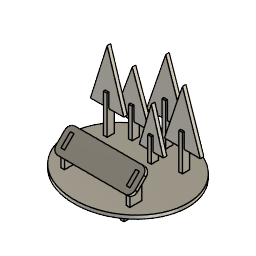
lasercutting v14 (Autodesk Fusion 360 design; units mm, degrees)
Autodesk Fusion 360 part; units mm, degrees
(part 1 of 2)
sketch "Sketch1" plane through (0, 0, 0) normal (0, 0, 1) x (1, 0, 0)
  circle A0 centre (0, 25) radius 50 construction
  ellipse E0 centre (0, 25) end of major axis (-50, 25) minor radius 45
  line L0 (50, 25) -> (-50, 25) construction
  line L1 (0, 70) -> (0, -20) construction
  dimension "d3" = 100
  constraint coincident E0 L0.start
  constraint coincident E0 L0.end
  constraint coincident E0 L1.start
  constraint coincident E0 L1.end
  constraint concentric A0 E0
  constraint horizontal L0
  measures "d3" diameter of A0
extrude "Extrude1" add sketch "Sketch1" along normal blind 3 makes body 1
sketch "Sketch2" plane through (0, 0, 3) normal (0, 0, 1) x (-1, 0, 0)
  line L0 (28.8477, -7.7401) -> (25.8477, -7.7401)
  line L1 (25.8477, -7.7401) -> (25.8477, 2.2599)
  line L2 (25.8477, 2.2599) -> (28.8477, 2.2599)
  line L3 (28.8477, 2.2599) -> (28.8477, -7.7401)
  line L4 (0, -100) -> (0, 100) construction
  line L5 (-28.8477, -7.7401) -> (-25.8477, -7.7401)
  line L6 (-25.8477, -7.7401) -> (-25.8477, 2.2599)
  line L7 (-28.8477, 2.2599) -> (-28.8477, -7.7401)
  line L8 (-25.8477, 2.2599) -> (-28.8477, 2.2599)
  ellipse E0 centre (0, -25) end of major axis (50, -25) minor radius 45
  dimension "d6" = 3
  constraint horizontal L0
  constraint vertical L1
  constraint horizontal L2
  constraint vertical L3
  constraint vertical L4
  constraint symmetric L0.start L4 L5.start
  constraint symmetric L0.end L4 L5.end
  constraint symmetric L1.end L4 L6.end
  constraint symmetric L2.end L4 L7.start
  measures "d6" distance of L0.start L0.end
extrude "Extrude2" add sketch "Sketch2" along normal blind 20 separate body contours L0 L1 L2 L3 | L5 L6 L7 L8 makes body 2 at (-25.8477, 4.4068, 9.6667) makes body 3 at (28.8477, 1.0734, 9.6667)
extrude "Extrude3" add sketch "Sketch2" against normal blind 8 contours L0 L1 L2 L3 | L5 L6 L7 L8 bodies 2 3
sketch "Sketch3" plane through (0, -2.2599, 0) normal (0, -1, 0) x (1, 0, 0)
  line L0 (-25.8477, -5) -> (-25.8477, 23)
  line L1 (-25.8477, 23) -> (-28.8477, 23)
  line L2 (-28.8477, 23) -> (-28.8477, -5)
  line L3 (-28.8477, -5) -> (-25.8477, -5)
  line L4 (0, 15) -> (0, -10) construction
  line L5 (-28.8477, 0.0164) -> (-25.8477, 0.0164)
  line L6 (-25.8477, 0.0164) -> (-25.8477, -5)
  line L7 (-25.8477, -5) -> (-28.8477, -5)
  line L8 (-28.8477, -5) -> (-28.8477, 0.0164)
  line L9 (28.8477, 0.0164) -> (25.8477, 0.0164)
  line L10 (28.8477, -5) -> (28.8477, 0.0164)
  line L11 (25.8477, -5) -> (28.8477, -5)
  line L12 (25.8477, 0.0164) -> (25.8477, -5)
  constraint vertical L4
  constraint horizontal L5
  constraint vertical L6
  constraint horizontal L7
  constraint vertical L8
  constraint coincident L0.start L3.end
  constraint coincident L2 L5.start
  constraint symmetric L4 L5.start L9.start
  constraint symmetric L4 L5.end L9.end
  constraint symmetric L4 L0.start L11.start
  constraint symmetric L4 L2.end L10.start
extrude "Extrude4" add sketch "Sketch3" along normal blind 5 contours L0 L2 L3 L5 L6 L7 L8 | L9 L10 L11 L12 bodies 2 3
extrude "Extrude5" add sketch "Sketch3" against normal blind 5 from surface at -10 contours L0 L2 L3 L5 L6 L7 L8 | L9 L10 L11 L12 bodies 2 3
chamfer "Chamfer1" distance 10 angle 45 2 edges at (27.3477, -2.2599, 23) (-27.3477, -2.2599, 23) on bodies 2 3
extrude "Extrude6" add 2 faces at (-26.8477, 7.7388, 23) (-26.8477, 1.0728, 16.3347) along direction (0, -0.707107, 0.707107) blind 3 separate body on bodies 2 makes body 4
move_face "OffsetFaces1" offset -3 1 faces at (-26.8477, -2.967, 13.7091) on bodies 4
mirror "Mirror1" about plane through (0, 0, 0) normal (1, 0, 0) of bodies 4 makes body 5
combine "Combine1" operation add target body 4 tool bodies 2 5 3 makes body 6 at (28.8477, 5.1139, 12.7132)
sketch "Sketch5" plane through (0, -9.7513, 9.7513) normal (0, -0.707107, 0.707107) x (1, 0, 0)
  line L0 (-25.8477, 10.5944) -> (-25.8477, 21.7365)
  line L1 (-25.8477, 21.7365) -> (-28.8477, 21.7365)
  line L2 (-28.8477, 21.7365) -> (-28.8477, 10.5944)
  line L3 (-28.8477, 10.5944) -> (-25.8477, 10.5944)
  line L4 (0, 4) -> (0, -46) construction
  line L5 (0, 25.9792) -> (0, 5.8372)
  line L6 (0, 5.8372) -> (-28, 5.8372)
  line L7 (-33, 10.8372) -> (-33, 20.9792)
  line L8 (-28, 25.9792) -> (0, 25.9792)
  arc A0 (-28, 25.9792) -> (-33, 20.9792) centre (-28, 20.9792) ccw
  arc A1 (-33, 10.8372) -> (-28, 5.8372) centre (-28, 10.8372) ccw
  dimension "d24" = 5
  constraint vertical L4
  constraint vertical L5
  constraint tangent L7 A0
  constraint tangent L8 A0
  constraint tangent L6 A1
  constraint tangent L7 A1
  constraint equal A0 A1
  measures "d24" radius of A0
extrude "Extrude7" add sketch "Sketch5" against normal blind 3 separate body makes body 7
mirror "Mirror2" about plane through (0, 0, 0) normal (1, 0, 0) of bodies 7 merged
sketch "Sketch6" plane through (0, 0, 3) normal (0, 0, 1) x (-1, 0, 0)
  line L0 (-1.5, -55) -> (1.5, -55)
  line L1 (1.5, -55) -> (1.5, -61)
  line L2 (1.5, -61) -> (-1.5, -61)
  line L3 (-1.5, -61) -> (-1.5, -55)
  line L4 (-1.5, -55) -> (1.5, -61) construction
  line L5 (1.5, -55) -> (-1.5, -61) construction
  line L6 (18.5, -47) -> (21.5, -47)
  line L7 (21.5, -47) -> (21.5, -53)
  line L8 (21.5, -53) -> (18.5, -53)
  line L9 (18.5, -53) -> (18.5, -47)
  line L10 (18.5, -47) -> (21.5, -53) construction
  line L11 (21.5, -47) -> (18.5, -53) construction
  line L12 (-23.5, -44) -> (-26.5, -44)
  line L13 (-26.5, -44) -> (-26.5, -50)
  line L14 (-26.5, -50) -> (-23.5, -50)
  line L15 (-23.5, -50) -> (-23.5, -44)
  line L16 (-23.5, -44) -> (-26.5, -50) construction
  line L17 (-26.5, -44) -> (-23.5, -50) construction
  line L18 (-6.5, -38) -> (-3.5, -38)
  line L19 (-3.5, -38) -> (-3.5, -44)
  line L20 (-3.5, -44) -> (-6.5, -44)
  line L21 (-6.5, -44) -> (-6.5, -38)
  line L22 (-6.5, -38) -> (-3.5, -44) construction
  line L23 (-3.5, -38) -> (-6.5, -44) construction
  line L24 (31.5, -39) -> (34.5, -39)
  line L25 (34.5, -39) -> (34.5, -45)
  line L26 (34.5, -45) -> (31.5, -45)
  line L27 (31.5, -45) -> (31.5, -39)
  line L28 (31.5, -39) -> (34.5, -45) construction
  line L29 (34.5, -39) -> (31.5, -45) construction
  ellipse E0 centre (0, -25) end of major axis (50, -25) minor radius 45
  point P0 (0, -58)
  point P1 (20, -50)
  point P2 (-25, -47)
  point P3 (-5, -41)
  point P4 (33, -42)
  dimension "d29" = 3
  dimension "d30" = 6
  dimension "d49" = 3
  dimension "d50" = 3
  dimension "d51" = 6
  dimension "d52" = 3
  dimension "d53" = 3
  dimension "d54" = 6
  constraint horizontal L0
  constraint perpendicular L0 L1
  constraint parallel L0 L2
  constraint parallel L1 L3
  constraint coincident L4 P0
  constraint coincident L5 P0
  constraint horizontal L6
  constraint perpendicular L6 L7
  constraint parallel L6 L8
  constraint parallel L7 L9
  constraint coincident L10 P1
  constraint coincident L11 P1
  constraint horizontal L12
  constraint perpendicular L12 L13
  constraint parallel L12 L14
  constraint parallel L13 L15
  constraint coincident L16 P2
  constraint coincident L17 P2
  constraint horizontal L18
  constraint perpendicular L18 L19
  constraint parallel L18 L20
  constraint parallel L19 L21
  constraint coincident L22 P3
  constraint coincident L23 P3
  constraint horizontal L24
  constraint perpendicular L24 L25
  constraint parallel L24 L26
  constraint parallel L25 L27
  constraint coincident L28 P4
  constraint coincident L29 P4
  measures "d29" distance of L1.end L2.end
  measures "d30" distance of L0.end L1.end
  measures "d49" distance of L7.end L8.end
  measures "d50" distance of L13.end L14.end
  measures "d51" distance of L12.end L13.end
  measures "d52" distance of L19.end L20.end
  measures "d53" distance of L25.end L26.end
  measures "d54" distance of L24.end L25.end
extrude "Extrude8" add sketch "Sketch6" along normal blind 35 separate body contours L0 L1 L2 L3 makes body 8
sketch "Sketch7" plane through (-1.5, 0, 0) normal (-1, 0, 0) x (0, -1, 0)
  line L0 (-55, 3) -> (-55, 38)
  line L1 (-55, 38) -> (-61, 38)
  line L2 (-61, 38) -> (-61, 3)
  line L3 (-59.5, 33) -> (-56.5, 33)
  line L4 (-56.5, 33) -> (-56.5, 43)
  line L5 (-56.5, 43) -> (-59.5, 43)
  line L6 (-59.5, 43) -> (-59.5, 33)
  line L7 (-59.5, 33) -> (-56.5, 43) construction
  line L8 (-56.5, 33) -> (-59.5, 43) construction
  line L9 (-61, 3) -> (-55, 3)
  point P0 (-58, 38)
  dimension "d33" = 3
  dimension "d34" = 10
  constraint horizontal L3
  constraint perpendicular L3 L4
  constraint parallel L3 L5
  constraint parallel L4 L6
  constraint coincident L7 P0
  constraint coincident L8 P0
  constraint midpoint L1 P0
  measures "d33" distance of L4.end L5.end
  measures "d34" distance of L3.end L4.end
extrude "Extrude9" cut sketch "Sketch7" against normal blind 3 contours L1 L3 L4 L6 bodies 1 8
extrude "Extrude10" add sketch "Sketch6" against normal blind 8 contours L0 L1 L2 L3 bodies 8
sketch "Sketch8" plane through (0, 61, 0) normal (0, 1, 0) x (-1, 0, 0)
  line L0 (1.5, -5) -> (1.5, 38)
  line L1 (1.5, 38) -> (-1.5, 38)
  line L2 (-1.5, 38) -> (-1.5, -5)
  line L3 (-1.5, -5) -> (1.5, -5)
  line L4 (-1.5, 0) -> (1.5, 0)
  line L5 (1.5, 0) -> (1.5, -5)
  line L6 (1.5, -5) -> (-1.5, -5)
  line L7 (-1.5, -5) -> (-1.5, 0)
  constraint horizontal L4
  constraint vertical L5
  constraint horizontal L6
  constraint vertical L7
  constraint coincident L0.start L3.end
  constraint coincident L2 L4.start
extrude "Extrude11" add sketch "Sketch8" along normal blind 5 contours L0 L2 L3 L4 L5 L6 L7 bodies 8
extrude "Extrude12" add sketch "Sketch8" against normal blind 11 contours L0 L2 L3 L4 L5 L6 L7 bodies 8
sketch "Sketch9" plane through (0, 59.5, 0) normal (0, -1, 0) x (1, 0, 0)
  line L0 (-1.5, 38) -> (-1.5, 33)
  line L1 (-1.5, 33) -> (1.5, 33)
  line L2 (1.5, 33) -> (1.5, 38)
  line L3 (1.5, 38) -> (-1.5, 38)
  line L4 (-6, 38) -> (5.5, 38) construction
  line L5 (-6.5, 33) -> (5.7756, 33) construction
  line L6 (0, 70) -> (-16.0582, 22.6488)
  line L7 (-1.5, 38) -> (-1.5, 16) construction
  line L8 (-16.0582, 22.6488) -> (-1.5, 22.6488)
  line L9 (-1.5, 33) -> (-1.5, 22.6488)
  line L10 (0, 85) -> (0, 0) construction
  line L11 (0, 70) -> (16.0582, 22.6488)
  line L12 (16.0582, 22.6488) -> (1.5, 22.6488)
  line L13 (1.5, 33) -> (1.5, 22.6488)
  line L14 (-1.5, 33) -> (1.5, 33)
  dimension "d45" = 5
  dimension "d46" = 50
  constraint perpendicular L2 L4
  constraint perpendicular L0 L5
  constraint coincident L0.start L3.end
  constraint perpendicular L5 L7
  constraint coincident L7 L8.end
  constraint perpendicular L7 L8
  constraint coincident L0.end L1.start
  constraint coincident L10.end origin
  constraint perpendicular L8 L10
  constraint symmetric L6.start L10 L11.start
  constraint symmetric L6.end L10 L11.end
  constraint symmetric L8.end L10 L12.end
  constraint symmetric L0.end L10 L1.end
  measures "d45" distance of L4 L5
  measures "d46" distance of L6.start L6.end
extrude "Extrude13" add sketch "Sketch9" along normal blind 3 separate body contours L0 L2 L3 L6 L8 L9 L11 L12 L13 makes body 9
extrude "Extrude14" add sketch "Sketch6" along normal blind 25 separate body contours L6 L7 L8 L9 makes body 10
extrude "Extrude15" add sketch "Sketch6" against normal blind 8 contours L6 L7 L8 L9 bodies 10
sketch "Sketch10" plane through (0, 47, 0) normal (0, -1, 0) x (1, 0, 0)
  line L0 (-18.5, -5) -> (-18.5, 28)
  line L1 (-18.5, 28) -> (-21.5, 28)
  line L2 (-21.5, 28) -> (-21.5, -5)
  line L3 (-21.5, -5) -> (-18.5, -5)
  line L4 (-21.5, 0) -> (-18.5, 0)
  line L5 (-18.5, 0) -> (-18.5, -5)
  line L6 (-18.5, -5) -> (-21.5, -5)
  line L7 (-21.5, -5) -> (-21.5, 0)
  constraint horizontal L4
  constraint vertical L5
  constraint horizontal L6
  constraint vertical L7
  constraint coincident L0.start L3.end
  constraint coincident L2 L4.start
extrude "Extrude16" add sketch "Sketch10" along normal blind 5 contours L0 L2 L3 L4 L5 L6 L7 bodies 10
extrude "Extrude17" add sketch "Sketch10" against normal blind 11 contours L0 L2 L3 L4 L5 L6 L7 bodies 10
sketch "Sketch11" plane through (-21.5, 0, 0) normal (-1, 0, 0) x (0, -1, 0)
  line L0 (-47, 0) -> (-47, 28)
  line L1 (-47, 28) -> (-53, 28)
  line L2 (-53, 28) -> (-53, 0)
  line L3 (-53, 0) -> (-58, 0)
  line L4 (-58, 0) -> (-58, -5)
  line L5 (-58, -5) -> (-42, -5)
  line L6 (-42, -5) -> (-42, 0)
  line L7 (-42, 0) -> (-47, 0)
  line L8 (-48.5, 33) -> (-51.5, 33)
  line L9 (-51.5, 33) -> (-51.5, 23)
  line L10 (-51.5, 23) -> (-48.5, 23)
  line L11 (-48.5, 23) -> (-48.5, 33)
  line L12 (-48.5, 33) -> (-51.5, 23) construction
  line L13 (-51.5, 33) -> (-48.5, 23) construction
  point P0 (-50, 28)
  dimension "d63" = 3
  dimension "d64" = 10
  constraint horizontal L8
  constraint perpendicular L8 L9
  constraint parallel L8 L10
  constraint parallel L9 L11
  constraint coincident L12 P0
  constraint coincident L13 P0
  constraint midpoint L1 P0
  measures "d63" distance of L9.end L10.end
  measures "d64" distance of L8.end L9.end
extrude "Extrude18" cut sketch "Sketch11" against normal blind 3 contours L1 L9 L10 L11 bodies 10
sketch "Sketch12" plane through (0, 51.5, 0) normal (0, -1, 0) x (1, 0, 0)
  line L0 (-21.5, 28) -> (-21.5, 23)
  line L1 (-21.5, 23) -> (-18.5, 23)
  line L2 (-18.5, 23) -> (-18.5, 28)
  line L3 (-18.5, 28) -> (-21.5, 28)
  line L4 (-24.1, 28) -> (-15.2, 28) construction
  line L5 (-23.9, 23) -> (-15.1, 23) construction
  line L6 (-20, 55) -> (-34, 16)
  line L7 (-21.5, 28) -> (-21.5, 10) construction
  line L8 (-34, 16) -> (-21.5, 16)
  line L9 (-21.5, 16) -> (-21.5, 23)
  line L10 (-21.5, 23) -> (-20, 23)
  line L11 (-20, 59) -> (-20, 5) construction
  line L12 (-20, 55) -> (-6, 16)
  line L13 (-6, 16) -> (-18.5, 16)
  line L14 (-18.5, 16) -> (-18.5, 23)
  line L15 (-18.5, 23) -> (-20, 23)
  dimension "d67" = 5
  constraint perpendicular L2 L4
  constraint perpendicular L2 L5
  constraint coincident L0.start L3.end
  constraint perpendicular L4 L7
  constraint coincident L7 L8.end
  constraint perpendicular L7 L8
  constraint coincident L0.end L1.start
  constraint midpoint L1 L10.end
  constraint perpendicular L10 L11
  constraint symmetric L6.start L11 L12.start
  constraint symmetric L6.end L11 L12.end
  constraint symmetric L8.end L11 L13.end
  constraint symmetric L0.end L11 L1.end
  constraint symmetric L10.end L11 L15.end
  measures "d67" distance of L4 L5
extrude "Extrude19" add sketch "Sketch12" along normal blind 3 separate body contours L0 L2 L3 L6 L8 L9 L12 L13 L14 makes body 11
extrude "Extrude20" add sketch "Sketch6" along normal blind 30 separate body contours L12 L13 L14 L15 makes body 12
extrude "Extrude21" add sketch "Sketch6" against normal blind 8 contours L12 L13 L14 L15 bodies 12
sketch "Sketch13" plane through (0, 44, 0) normal (0, -1, 0) x (1, 0, 0)
  line L0 (26.5, -5) -> (26.5, 33)
  line L1 (26.5, 33) -> (23.5, 33)
  line L2 (23.5, 33) -> (23.5, -5)
  line L3 (23.5, -5) -> (26.5, -5)
  line L4 (23.5, 0) -> (26.5, 0)
  line L5 (26.5, 0) -> (26.5, -5)
  line L6 (26.5, -5) -> (23.5, -5)
  line L7 (23.5, -5) -> (23.5, 0)
  constraint horizontal L4
  constraint vertical L5
  constraint horizontal L6
  constraint vertical L7
  constraint coincident L0.start L3.end
  constraint coincident L2 L4.start
extrude "Extrude22" add sketch "Sketch13" along normal blind 5 contours L0 L2 L3 L4 L5 L6 L7 bodies 12
extrude "Extrude23" add sketch "Sketch13" against normal blind 11 contours L0 L2 L3 L4 L5 L6 L7 bodies 12
sketch "Sketch14" plane through (26.5, 0, 0) normal (1, 0, 0) x (0, 1, 0)
  line L0 (50, 0) -> (50, 33)
  line L1 (50, 33) -> (44, 33)
  line L2 (44, 33) -> (44, 0)
  line L3 (44, 0) -> (39, 0)
  line L4 (39, 0) -> (39, -5)
  line L5 (39, -5) -> (55, -5)
  line L6 (55, -5) -> (55, 0)
  line L7 (55, 0) -> (50, 0)
  line L8 (45.5, 28) -> (48.5, 28)
  line L9 (48.5, 28) -> (48.5, 38)
  line L10 (48.5, 38) -> (45.5, 38)
  line L11 (45.5, 38) -> (45.5, 28)
  line L12 (45.5, 28) -> (48.5, 38) construction
  line L13 (48.5, 28) -> (45.5, 38) construction
  point P0 (47, 33)
  dimension "d78" = 3
  dimension "d79" = 10
  constraint horizontal L8
  constraint perpendicular L8 L9
  constraint parallel L8 L10
  constraint parallel L9 L11
  constraint coincident L12 P0
  constraint coincident L13 P0
  constraint midpoint L1 P0
  measures "d78" distance of L9.end L10.end
  measures "d79" distance of L8.end L9.end
extrude "Extrude24" cut sketch "Sketch14" against normal blind 3 contours L1 L8 L9 L11 bodies 12
sketch "Sketch15" plane through (0, 48.5, 0) normal (0, -1, 0) x (1, 0, 0)
  line L0 (26.5, 28) -> (26.5, 33)
  line L1 (26.5, 33) -> (23.5, 33)
  line L2 (23.5, 33) -> (23.5, 28)
  line L3 (23.5, 28) -> (26.5, 28)
  line L4 (20.7463, 33) -> (31.5, 33) construction
  line L5 (20.7463, 28) -> (31.5, 28) construction
  line L6 (23.5, 35) -> (23.5, 13) construction
  line L7 (25, 57) -> (25, 12) construction
  line L8 (25, 65) -> (10, 20)
  line L9 (10, 20) -> (23.5, 20)
  line L10 (23.5, 20) -> (23.5, 28)
  line L11 (23.5, 28) -> (25, 28)
  line L12 (25, 65) -> (40, 20)
  line L13 (40, 20) -> (26.5, 20)
  line L14 (26.5, 20) -> (26.5, 28)
  line L15 (26.5, 28) -> (25, 28)
  dimension "d82" = 5
  constraint perpendicular L0 L4
  constraint parallel L4 L5
  constraint perpendicular L5 L6
  constraint perpendicular L5 L7
  constraint coincident L6 L9.end
  constraint perpendicular L6 L9
  constraint coincident L2.end L3.start
  constraint midpoint L3 L11.end
  constraint symmetric L7 L8.start L12.start
  constraint symmetric L7 L8.end L12.end
  constraint symmetric L7 L9.end L13.end
  constraint symmetric L7 L2.end L0.start
  constraint symmetric L7 L11.end L15.end
  measures "d82" distance of L4 L5
extrude "Extrude25" add sketch "Sketch15" along normal blind 3 separate body contours L0 L1 L2 L8 L9 L10 L12 L13 L14 makes body 13
extrude "Extrude26" add sketch "Sketch6" along normal blind 32 separate body contours L24 L25 L26 L27 makes body 14
extrude "Extrude27" add sketch "Sketch6" against normal blind 8 contours L24 L25 L26 L27 bodies 14
sketch "Sketch16" plane through (0, 39, 0) normal (0, -1, 0) x (1, 0, 0)
  line L0 (-31.5, -5) -> (-31.5, 35)
  line L1 (-31.5, 35) -> (-34.5, 35)
  line L2 (-34.5, 35) -> (-34.5, -5)
  line L3 (-34.5, -5) -> (-31.5, -5)
  line L4 (-34.5, 0) -> (-31.5, 0)
  line L5 (-31.5, 0) -> (-31.5, -5)
  line L6 (-31.5, -5) -> (-34.5, -5)
  line L7 (-34.5, -5) -> (-34.5, 0)
  constraint horizontal L4
  constraint vertical L5
  constraint horizontal L6
  constraint vertical L7
  constraint coincident L0.start L3.end
  constraint coincident L2 L4.start
extrude "Extrude28" add sketch "Sketch16" along normal blind 5 contours L0 L2 L3 L4 L5 L6 L7 bodies 14
extrude "Extrude29" add sketch "Sketch16" against normal blind 11 contours L0 L2 L3 L4 L5 L6 L7 bodies 14
sketch "Sketch17" plane through (-34.5, 0, 0) normal (-1, 0, 0) x (0, -1, 0)
  line L0 (-39, 0) -> (-39, 35)
  line L1 (-39, 35) -> (-45, 35)
  line L2 (-45, 35) -> (-45, 0)
  line L3 (-45, 0) -> (-50, 0)
  line L4 (-50, 0) -> (-50, -5)
  line L5 (-50, -5) -> (-34, -5)
  line L6 (-34, -5) -> (-34, 0)
  line L7 (-34, 0) -> (-39, 0)
  line L8 (-40.5, 40) -> (-43.5, 40)
  line L9 (-43.5, 40) -> (-43.5, 30)
  line L10 (-43.5, 30) -> (-40.5, 30)
  line L11 (-40.5, 30) -> (-40.5, 40)
  line L12 (-40.5, 40) -> (-43.5, 30) construction
  line L13 (-43.5, 40) -> (-40.5, 30) construction
  point P0 (-42, 35)
  dimension "d93" = 3
  dimension "d94" = 10
  constraint horizontal L8
  constraint perpendicular L8 L9
  constraint parallel L8 L10
  constraint parallel L9 L11
  constraint coincident L12 P0
  constraint coincident L13 P0
  constraint midpoint L1 P0
  measures "d93" distance of L9.end L10.end
  measures "d94" distance of L8.end L9.end
extrude "Extrude30" cut sketch "Sketch17" against normal blind 3 contours L1 L9 L10 L11 bodies 14
sketch "Sketch18" plane through (0, 43.5, 0) normal (0, -1, 0) x (1, 0, 0)
  line L0 (-34.5, 35) -> (-34.5, 30)
  line L1 (-34.5, 30) -> (-31.5, 30)
  line L2 (-31.5, 30) -> (-31.5, 35)
  line L3 (-31.5, 35) -> (-34.5, 35)
  line L4 (-38, 35) -> (-29, 35) construction
  line L5 (-38.4345, 30) -> (-28.5, 30) construction
  line L6 (-34.5, 36.4776) -> (-34.5, 15.5578) construction
  line L7 (-33, 73) -> (-33, 8) construction
  line L8 (-33, 68) -> (-47, 23)
  line L9 (-47, 23) -> (-34.5, 23)
  line L10 (-34.5, 23) -> (-34.5, 30)
  line L11 (-34.5, 30) -> (-33, 30)
  line L12 (-33, 68) -> (-19, 23)
  line L13 (-19, 23) -> (-31.5, 23)
  line L14 (-31.5, 23) -> (-31.5, 30)
  line L15 (-31.5, 30) -> (-33, 30)
  dimension "d97" = 5
  constraint perpendicular L0 L4
  constraint horizontal L5
  constraint perpendicular L5 L6
  constraint perpendicular L5 L7
  constraint coincident L7 L8.start
  constraint coincident L6 L9.end
  constraint perpendicular L6 L9
  constraint coincident L0.end L1.start
  constraint perpendicular L5 L10
  constraint midpoint L1 L11.end
  constraint symmetric L7 L8.start L12.start
  constraint symmetric L7 L8.end L12.end
  constraint symmetric L7 L9.end L13.end
  constraint symmetric L7 L0.end L1.end
  constraint symmetric L7 L11.end L15.end
  measures "d97" distance of L4 L5
extrude "Extrude31" add sketch "Sketch18" along normal blind 3 separate body contours L0 L2 L3 L8 L9 L10 L12 L13 L14 makes body 15
extrude "Extrude32" add sketch "Sketch6" along normal blind 20 separate body contours L18 L19 L20 L21 makes body 16
extrude "Extrude33" add sketch "Sketch6" against normal blind 8 contours L18 L19 L20 L21 bodies 16
sketch "Sketch19" plane through (0, 38, 0) normal (0, -1, 0) x (1, 0, 0)
  line L0 (6.5, -5) -> (6.5, 23)
  line L1 (6.5, 23) -> (3.5, 23)
  line L2 (3.5, 23) -> (3.5, -5)
  line L3 (3.5, -5) -> (6.5, -5)
  line L4 (3.5, 0) -> (6.5, 0)
  line L5 (6.5, 0) -> (6.5, -5)
  line L6 (6.5, -5) -> (3.5, -5)
  line L7 (3.5, -5) -> (3.5, 0)
  constraint horizontal L4
  constraint vertical L5
  constraint horizontal L6
  constraint vertical L7
  constraint coincident L0.start L3.end
  constraint coincident L2 L4.start
extrude "Extrude34" add sketch "Sketch19" along normal blind 5 contours L0 L2 L3 L4 L5 L6 L7 bodies 16
extrude "Extrude35" add sketch "Sketch19" against normal blind 11 contours L0 L2 L3 L4 L5 L6 L7 bodies 16
sketch "Sketch20" plane through (6.5, 0, 0) normal (1, 0, 0) x (0, 1, 0)
  line L0 (44, 0) -> (44, 23)
  line L1 (44, 23) -> (38, 23)
  line L2 (38, 23) -> (38, 0)
  line L3 (38, 0) -> (33, 0)
  line L4 (33, 0) -> (33, -5)
  line L5 (33, -5) -> (49, -5)
  line L6 (49, -5) -> (49, 0)
  line L7 (49, 0) -> (44, 0)
  line L8 (39.5, 18) -> (42.5, 18)
  line L9 (42.5, 18) -> (42.5, 28)
  line L10 (42.5, 28) -> (39.5, 28)
  line L11 (39.5, 28) -> (39.5, 18)
  line L12 (39.5, 18) -> (42.5, 28) construction
  line L13 (42.5, 18) -> (39.5, 28) construction
  point P0 (41, 23)
  dimension "d108" = 3
  dimension "d109" = 10
  constraint horizontal L8
  constraint perpendicular L8 L9
  constraint parallel L8 L10
  constraint parallel L9 L11
  constraint coincident L12 P0
  constraint coincident L13 P0
  constraint midpoint L1 P0
  measures "d108" distance of L9.end L10.end
  measures "d109" distance of L8.end L9.end
extrude "Extrude36" cut sketch "Sketch20" against normal blind 3 contours L1 L8 L9 L11 bodies 16
sketch "Sketch21" plane through (0, 42.5, 0) normal (0, -1, 0) x (1, 0, 0)
  line L0 (6.5, 18) -> (6.5, 23)
  line L1 (6.5, 23) -> (3.5, 23)
  line L2 (3.5, 23) -> (3.5, 18)
  line L3 (3.5, 18) -> (6.5, 18)
  line L4 (1.5, 23) -> (12.5, 23) construction
  line L5 (3.5, 28.0693) -> (3.5, 5) construction
  line L6 (5, 68.4762) -> (5, -10) construction
  line L7 (5, 45) -> (-5, 11)
  line L8 (-5, 11) -> (3.5, 11)
  line L9 (3.5, 11) -> (3.5, 18)
  line L10 (3.5, 18) -> (5, 18)
  line L11 (5, 45) -> (15, 11)
  line L12 (6.5, 11) -> (6.5, 18)
  line L13 (6.5, 18) -> (5, 18)
  line L14 (15, 11) -> (6.5, 11)
  constraint perpendicular L2 L4
  constraint perpendicular L1 L5
  constraint coincident L6 L7.start
  constraint coincident L5 L8.end
  constraint perpendicular L5 L8
  constraint coincident L2.end L3.start
  constraint midpoint L3 L10.end
  constraint symmetric L6 L7.start L11.start
  constraint symmetric L6 L7.end L11.end
  constraint symmetric L6 L8.end L12.start
  constraint symmetric L6 L2.end L0.start
  constraint symmetric L6 L10.end L13.end
extrude "Extrude37" add sketch "Sketch21" along normal blind 3 separate body contours L0 L1 L2 L7 L8 L9 L11 L12 L14 makes body 17
extrude "Extrude38" cut sketch "Sketch6" against normal blind 3 contours L0 L1 L2 L3 | L6 L7 L8 L9 | L12 L13 L14 L15 | L18 L19 L20 L21 | L24 L25 L26 L27 bodies 1
extrude "Extrude39" cut sketch "Sketch2" against normal blind 3 contours L0 L1 L2 L3 | L5 L6 L7 L8 bodies 1
sketch "Sketch22" plane through (0, 0, 3) normal (0, 0, 1) x (-1, 0, 0)
  line L0 (25.8477, -7.7401) -> (25.8477, 2.2599)
  line L1 (25.8477, 2.2599) -> (28.8477, 2.2599)
  line L2 (28.8477, 2.2599) -> (28.8477, -7.7401) construction
  line L3 (28.8477, -7.7401) -> (25.8477, -7.7401)
  line L4 (-28.8477, -7.7401) -> (-28.8477, 2.2599)
  line L5 (-28.8477, 2.2599) -> (-25.8477, 2.2599)
  line L6 (-25.8477, 2.2599) -> (-25.8477, -7.7401) construction
  line L7 (-25.8477, -7.7401) -> (-28.8477, -7.7401)
  line L8 (1.5, -55) -> (1.5, -61) construction
  line L9 (1.5, -61) -> (-1.5, -61)
  line L10 (-1.5, -61) -> (-1.5, -55)
  line L11 (-1.5, -55) -> (1.5, -55)
  line L12 (21.5, -47) -> (21.5, -53) construction
  line L13 (21.5, -53) -> (18.5, -53)
  line L14 (18.5, -53) -> (18.5, -47)
  line L15 (18.5, -47) -> (21.5, -47)
  line L16 (-3.5, -38) -> (-3.5, -44) construction
  line L17 (-3.5, -44) -> (-6.5, -44)
  line L18 (-6.5, -44) -> (-6.5, -38) construction
  line L19 (-6.5, -38) -> (-3.5, -38)
  line L20 (34.5, -39) -> (34.5, -45)
  line L21 (34.5, -45) -> (31.5, -45)
  line L22 (31.5, -45) -> (31.5, -39) construction
  line L23 (31.5, -39) -> (34.5, -39)
  line L24 (-26.5, -44) -> (-23.5, -44)
  line L25 (-23.5, -44) -> (-23.5, -50) construction
  line L26 (-23.5, -50) -> (-26.5, -50)
  line L27 (-26.5, -50) -> (-26.5, -44)
  ellipse E0 centre (0, -25) end of major axis (50, -25) minor radius 45
  spline S0 degree 3 poles (-50.15, -25) (-50.15, -32.5631) (-47.9958, -40.118) (-43.9509, -46.7448) (-39.8574, -53.4511) (-33.836, -59.192) (-26.6367, -63.255) (-19.363, -67.3601) (-10.9028, -69.7425) (-2.3285, -70.1013) (6.2391, -70.4598) (14.9013, -68.7971) (22.562, -65.3229) (30.4835, -61.7304) (37.313, -56.2069) (42.1269, -49.4968) (46.6731, -43.1599) (49.4152, -35.7814) (50.0195, -28.2553) (50.6245, -20.7198) (49.0848, -13.0525) (45.5885, -6.1855) (42.0575, 0.7493) (36.5382, 6.8528) (29.7144, 11.3714) (22.8186, 15.9376) (14.6055, 18.8748) (6.1105, 19.8136) (-2.4147, 20.7558) (-11.2046, 19.683) (-19.144, 16.731) (-26.9932, 13.8125) (-33.994, 9.0643) (-39.2761, 3.0748) (-44.4865, -2.8334) (-48.014, -9.9366) (-49.4296, -17.3744) (-49.9087, -19.8918) (-50.15, -22.4459) (-50.15, -25) knots -3.141593 -3.141593 -3.141593 -3.141593 -2.639249 -2.639249 -2.639249 -2.130883 -2.130883 -2.130883 -1.617258 -1.617258 -1.617258 -1.10403 -1.10403 -1.10403 -0.573327 -0.573327 -0.573327 -0.072137 -0.072137 -0.072137 0.429687 0.429687 0.429687 0.936474 0.936474 0.936474 1.448612 1.448612 1.448612 1.962576 1.962576 1.962576 2.470707 2.470707 2.470707 2.971946 2.971946 2.971946 3.141593 3.141593 3.141593 3.141593
  line L28 (34.35, -39.15) -> (34.35, -44.85)
  line L29 (34.35, -44.85) -> (31.65, -44.85)
  line L30 (31.65, -44.85) -> (31.65, -39.15)
  line L31 (31.65, -39.15) -> (34.35, -39.15)
  line L32 (18.65, -52.85) -> (18.65, -47.15)
  line L33 (18.65, -47.15) -> (21.35, -47.15)
  line L34 (21.35, -47.15) -> (21.35, -52.85)
  line L35 (21.35, -52.85) -> (18.65, -52.85)
  line L36 (-1.35, -60.85) -> (-1.35, -55.15)
  line L37 (-1.35, -55.15) -> (1.35, -55.15)
  line L38 (1.35, -55.15) -> (1.35, -60.85)
  line L39 (1.35, -60.85) -> (-1.35, -60.85)
  line L40 (-6.35, -43.85) -> (-6.35, -38.15)
  line L41 (-6.35, -38.15) -> (-3.65, -38.15)
  line L42 (-3.65, -38.15) -> (-3.65, -43.85)
  line L43 (-3.65, -43.85) -> (-6.35, -43.85)
  line L44 (-26.35, -49.85) -> (-26.35, -44.15)
  line L45 (-26.35, -44.15) -> (-23.65, -44.15)
  line L46 (-23.65, -44.15) -> (-23.65, -49.85)
  line L47 (-23.65, -49.85) -> (-26.35, -49.85)
  line L48 (25.9977, -7.5901) -> (25.9977, 2.1099)
  line L49 (25.9977, 2.1099) -> (28.6977, 2.1099)
  line L50 (28.6977, 2.1099) -> (28.6977, -7.5901)
  line L51 (28.6977, -7.5901) -> (25.9977, -7.5901)
  line L52 (-28.6977, -7.5901) -> (-28.6977, 2.1099)
  line L53 (-28.6977, 2.1099) -> (-25.9977, 2.1099)
  line L54 (-25.9977, 2.1099) -> (-25.9977, -7.5901)
  line L55 (-25.9977, -7.5901) -> (-28.6977, -7.5901)
  dimension "d119" = 0.15
  dimension "d120" = 0.15
  dimension "d121" = 0.15
  dimension "d122" = 0.15
  dimension "d123" = 0.15
  dimension "d124" = 0.15
  dimension "d125" = 0.15
  dimension "d126" = 0.15
sketch "Sketch23" plane through (-28.8477, 0, 0) normal (-1, 0, 0) x (0, -1, 0)
  line L0 (0.1386, 15.1213) -> (2.2599, 17.2426)
  line L1 (2.2599, 17.2426) -> (-5.6188, 25.1213)
  line L2 (-5.6188, 25.1213) -> (-7.7401, 23)
  line L3 (-7.7401, 23) -> (-7.7401, 0.0164)
  line L4 (-7.7401, 0.0164) -> (-12.7401, 0.0164)
  line L5 (-12.7401, 0.0164) -> (-12.7401, -5)
  line L6 (-12.7401, -5) -> (7.2599, -5)
  line L7 (7.2599, -5) -> (7.2599, 0.0164)
  line L8 (7.2599, 0.0164) -> (2.2599, 0.0164)
  line L9 (2.2599, 0.0164) -> (2.2599, 13)
  line L10 (2.2599, 13) -> (0.1386, 15.1213) construction
  line L11 (-7.8901, 23.0621) -> (-7.8901, 0.1664)
  line L12 (-7.8901, 0.1664) -> (-12.8901, 0.1664)
  line L13 (-12.8901, 0.1664) -> (-12.8901, -5.15)
  line L14 (-12.8901, -5.15) -> (7.4099, -5.15)
  line L15 (7.4099, -5.15) -> (7.4099, 0.1664)
  line L16 (7.4099, 0.1664) -> (2.4099, 0.1664)
  line L17 (2.4099, 0.1664) -> (2.4099, 13.0621)
  line L18 (2.4099, 13.0621) -> (0.3507, 15.1213)
  line L19 (0.3507, 15.1213) -> (2.472, 17.2426)
  line L20 (2.472, 17.2426) -> (-5.6188, 25.3335)
  line L21 (-5.6188, 25.3335) -> (-7.8901, 23.0621)
  dimension "d127" = 0.15
sketch "Sketch24" plane through (0, -9.7513, 9.7513) normal (0, -0.707107, 0.707107) x (1, 0, 0)
  line L0 (28.8477, 10.5944) -> (25.8477, 10.5944)
  line L1 (25.8477, 10.5944) -> (25.8477, 21.7365) construction
  line L2 (25.8477, 21.7365) -> (28.8477, 21.7365)
  line L3 (28.8477, 21.7365) -> (28.8477, 10.5944)
  line L4 (-25.8477, 10.5944) -> (-28.8477, 10.5944)
  line L5 (-28.8477, 10.5944) -> (-28.8477, 21.7365)
  line L6 (-28.8477, 21.7365) -> (-25.8477, 21.7365)
  line L7 (-25.8477, 21.7365) -> (-25.8477, 10.5944) construction
  arc A0 (-28, 25.9792) -> (-33, 20.9792) centre (-28, 20.9792) ccw
  line L8 (-33, 20.9792) -> (-33, 10.8372)
  arc A1 (-33, 10.8372) -> (-28, 5.8372) centre (-28, 10.8372) ccw
  line L9 (-28, 5.8372) -> (28, 5.8372)
  arc A2 (28, 5.8372) -> (33, 10.8372) centre (28, 10.8372) ccw
  line L10 (33, 10.8372) -> (33, 20.9792)
  arc A3 (33, 20.9792) -> (28, 25.9792) centre (28, 20.9792) ccw
  line L11 (28, 25.9792) -> (-28, 25.9792) construction
  line L12 (-33.15, 20.9792) -> (-33.15, 10.8372)
  arc A4 (-33.15, 10.8372) -> (-28, 5.6872) centre (-28, 10.8372) ccw
  line L13 (-28, 5.6872) -> (28, 5.6872)
  arc A5 (28, 5.6872) -> (33.15, 10.8372) centre (28, 10.8372) ccw
  line L14 (33.15, 10.8372) -> (33.15, 20.9792)
  arc A6 (33.15, 20.9792) -> (28, 26.1292) centre (28, 20.9792) ccw
  line L15 (28, 26.1292) -> (-28, 26.1292)
  arc A7 (-28, 26.1292) -> (-33.15, 20.9792) centre (-28, 20.9792) ccw
  line L16 (-25.9977, 21.5865) -> (-25.9977, 10.7444)
  line L17 (-25.9977, 10.7444) -> (-28.6977, 10.7444)
  line L18 (-28.6977, 10.7444) -> (-28.6977, 21.5865)
  line L19 (-28.6977, 21.5865) -> (-25.9977, 21.5865)
  line L20 (28.6977, 21.5865) -> (28.6977, 10.7444)
  line L21 (28.6977, 10.7444) -> (25.9977, 10.7444)
  line L22 (25.9977, 10.7444) -> (25.9977, 21.5865)
  line L23 (25.9977, 21.5865) -> (28.6977, 21.5865)
  dimension "d128" = 0.15
  dimension "d129" = 0.15
  dimension "d130" = 0.15
sketch "Sketch25" plane through (-1.5, 0, 0) normal (-1, 0, 0) x (0, -1, 0)
  line L0 (-55, 0) -> (-55, 38) construction
  line L1 (-55, 38) -> (-56.5, 38)
  line L2 (-56.5, 38) -> (-56.5, 33)
  line L3 (-56.5, 33) -> (-59.5, 33)
  line L4 (-59.5, 33) -> (-59.5, 38)
  line L5 (-59.5, 38) -> (-61, 38)
  line L6 (-61, 38) -> (-61, 0)
  line L7 (-61, 0) -> (-66, 0)
  line L8 (-66, 0) -> (-66, -5)
  line L9 (-66, -5) -> (-50, -5)
  line L10 (-50, -5) -> (-50, 0)
  line L11 (-50, 0) -> (-55, 0)
  line L12 (-56.65, 38.15) -> (-56.65, 33.15)
  line L13 (-56.65, 33.15) -> (-59.35, 33.15)
  line L14 (-59.35, 33.15) -> (-59.35, 38.15)
  line L15 (-59.35, 38.15) -> (-61.15, 38.15)
  line L16 (-61.15, 38.15) -> (-61.15, 0.15)
  line L17 (-61.15, 0.15) -> (-66.15, 0.15)
  line L18 (-66.15, 0.15) -> (-66.15, -5.15)
  line L19 (-66.15, -5.15) -> (-49.85, -5.15)
  line L20 (-49.85, -5.15) -> (-49.85, 0.15)
  line L21 (-49.85, 0.15) -> (-54.85, 0.15)
  line L22 (-54.85, 0.15) -> (-54.85, 38.15)
  line L23 (-54.85, 38.15) -> (-56.65, 38.15)
  dimension "d131" = 0.15
sketch "Sketch26" plane through (0, 56.5, 0) normal (0, -1, 0) x (1, 0, 0)
  line L0 (1.5, 38) -> (1.5, 22.6488)
  line L1 (1.5, 22.6488) -> (16.0582, 22.6488)
  line L2 (16.0582, 22.6488) -> (0, 70)
  line L3 (0, 70) -> (-16.0582, 22.6488)
  line L4 (-16.0582, 22.6488) -> (-1.5, 22.6488)
  line L5 (-1.5, 22.6488) -> (-1.5, 38)
  line L6 (-1.5, 38) -> (1.5, 38) construction
  line L7 (-1.35, 22.4988) -> (-1.35, 37.85)
  line L8 (-1.35, 37.85) -> (1.35, 37.85)
  line L9 (1.35, 37.85) -> (1.35, 22.4988)
  line L10 (1.35, 22.4988) -> (16.2675, 22.4988)
  line L11 (16.2675, 22.4988) -> (0, 70.4671)
  line L12 (0, 70.4671) -> (-16.2675, 22.4988)
  line L13 (-16.2675, 22.4988) -> (-1.35, 22.4988)
  dimension "d132" = 0.15
sketch "Sketch27" plane through (-21.5, 0, 0) normal (-1, 0, 0) x (0, -1, 0)
  line L0 (-48.5, 28) -> (-48.5, 23)
  line L1 (-48.5, 23) -> (-51.5, 23)
  line L2 (-51.5, 23) -> (-51.5, 28)
  line L3 (-51.5, 28) -> (-53, 28)
  line L4 (-53, 28) -> (-53, 0) construction
  line L5 (-53, 0) -> (-58, 0)
  line L6 (-58, 0) -> (-58, -5)
  line L7 (-58, -5) -> (-42, -5)
  line L8 (-42, -5) -> (-42, 0)
  line L9 (-42, 0) -> (-47, 0)
  line L10 (-47, 0) -> (-47, 28)
  line L11 (-47, 28) -> (-48.5, 28)
  line L12 (-58.15, 0.15) -> (-58.15, -5.15)
  line L13 (-58.15, -5.15) -> (-41.85, -5.15)
  line L14 (-41.85, -5.15) -> (-41.85, 0.15)
  line L15 (-41.85, 0.15) -> (-46.85, 0.15)
  line L16 (-46.85, 0.15) -> (-46.85, 28.15)
  line L17 (-46.85, 28.15) -> (-48.65, 28.15)
  line L18 (-48.65, 28.15) -> (-48.65, 23.15)
  line L19 (-48.65, 23.15) -> (-51.35, 23.15)
  line L20 (-51.35, 23.15) -> (-51.35, 28.15)
  line L21 (-51.35, 28.15) -> (-53.15, 28.15)
  line L22 (-53.15, 28.15) -> (-53.15, 0.15)
  line L23 (-53.15, 0.15) -> (-58.15, 0.15)
  dimension "d133" = 0.15
sketch "Sketch28" plane through (0, 48.5, 0) normal (0, -1, 0) x (1, 0, 0)
  line L0 (-20, 55) -> (-34, 16) construction
  line L1 (-34, 16) -> (-21.5, 16)
  line L2 (-21.5, 16) -> (-21.5, 28)
  line L3 (-21.5, 28) -> (-18.5, 28)
  line L4 (-18.5, 28) -> (-18.5, 16)
  line L5 (-18.5, 16) -> (-6, 16)
  line L6 (-6, 16) -> (-20, 55)
  line L7 (-21.35, 15.85) -> (-21.35, 27.85)
  line L8 (-21.35, 27.85) -> (-18.65, 27.85)
  line L9 (-18.65, 27.85) -> (-18.65, 15.85)
  line L10 (-18.65, 15.85) -> (-5.7868, 15.85)
  line L11 (-5.7868, 15.85) -> (-20, 55.444)
  line L12 (-20, 55.444) -> (-34.2132, 15.85)
  line L13 (-34.2132, 15.85) -> (-21.35, 15.85)
  dimension "d134" = 0.15
sketch "Sketch29" plane through (23.5, 0, 0) normal (-1, 0, 0) x (0, -1, 0)
  line L0 (-48.5, 28) -> (-48.5, 33) construction
  line L1 (-48.5, 33) -> (-50, 33) construction
  line L2 (-50, 33) -> (-50, 0) construction
  line L3 (-50, 0) -> (-55, 0) construction
  line L4 (-55, 0) -> (-55, -5) construction
  line L5 (-55, -5) -> (-39, -5) construction
  line L6 (-39, -5) -> (-39, 0) construction
  line L7 (-39, 0) -> (-44, 0) construction
  line L8 (-44, 0) -> (-44, 33) construction
  line L9 (-44, 33) -> (-45.5, 33) construction
  line L10 (-45.5, 33) -> (-45.5, 28) construction
  line L11 (-45.5, 28) -> (-48.5, 28) construction
  line L12 (-55.15, 0.15) -> (-55.15, -5.15)
  line L13 (-55.15, -5.15) -> (-38.85, -5.15)
  line L14 (-38.85, -5.15) -> (-38.85, 0.15)
  line L15 (-38.85, 0.15) -> (-43.85, 0.15)
  line L16 (-43.85, 0.15) -> (-43.85, 33.15)
  line L17 (-43.85, 33.15) -> (-45.65, 33.15)
  line L18 (-45.65, 33.15) -> (-45.65, 28.15)
  line L19 (-45.65, 28.15) -> (-48.35, 28.15)
  line L20 (-48.35, 28.15) -> (-48.35, 33.15)
  line L21 (-48.35, 33.15) -> (-50.15, 33.15)
  line L22 (-50.15, 33.15) -> (-50.15, 0.15)
  line L23 (-50.15, 0.15) -> (-55.15, 0.15)
  dimension "d135" = 0.15
sketch "Sketch30" plane through (0, 45.5, 0) normal (0, -1, 0) x (1, 0, 0)
  line L0 (25, 65) -> (10, 20) construction
  line L1 (10, 20) -> (23.5, 20)
  line L2 (23.5, 20) -> (23.5, 28)
  line L3 (23.5, 28) -> (23.5, 33)
  line L4 (23.5, 33) -> (26.5, 33)
  line L5 (26.5, 33) -> (26.5, 28)
  line L6 (26.5, 28) -> (26.5, 20)
  line L7 (26.5, 20) -> (40, 20)
  line L8 (40, 20) -> (25, 65)
  line L9 (23.65, 19.85) -> (23.65, 28)
  line L10 (23.65, 28) -> (23.65, 32.85)
  line L11 (23.65, 32.85) -> (26.35, 32.85)
  line L12 (26.35, 32.85) -> (26.35, 28)
  line L13 (26.35, 28) -> (26.35, 19.85)
  line L14 (26.35, 19.85) -> (40.2081, 19.85)
  line L15 (40.2081, 19.85) -> (25, 65.4743)
  line L16 (25, 65.4743) -> (9.7919, 19.85)
  line L17 (9.7919, 19.85) -> (23.65, 19.85)
  dimension "d136" = 0.15
sketch "Sketch31" plane through (-34.5, 0, 0) normal (-1, 0, 0) x (0, -1, 0)
  line L0 (-40.5, 35) -> (-40.5, 30)
  line L1 (-40.5, 30) -> (-43.5, 30)
  line L2 (-43.5, 30) -> (-43.5, 35)
  line L3 (-43.5, 35) -> (-45, 35)
  line L4 (-45, 35) -> (-45, 0)
  line L5 (-45, 0) -> (-50, 0)
  line L6 (-50, 0) -> (-50, -5)
  line L7 (-50, -5) -> (-34, -5)
  line L8 (-34, -5) -> (-34, 0)
  line L9 (-34, 0) -> (-39, 0)
  line L10 (-39, 0) -> (-39, 35) construction
  line L11 (-39, 35) -> (-40.5, 35)
  line L12 (-50.15, 0.15) -> (-50.15, -5.15)
  line L13 (-50.15, -5.15) -> (-33.85, -5.15)
  line L14 (-33.85, -5.15) -> (-33.85, 0.15)
  line L15 (-33.85, 0.15) -> (-38.85, 0.15)
  line L16 (-38.85, 0.15) -> (-38.85, 35.15)
  line L17 (-38.85, 35.15) -> (-40.65, 35.15)
  line L18 (-40.65, 35.15) -> (-40.65, 30.15)
  line L19 (-40.65, 30.15) -> (-43.35, 30.15)
  line L20 (-43.35, 30.15) -> (-43.35, 35.15)
  line L21 (-43.35, 35.15) -> (-45.15, 35.15)
  line L22 (-45.15, 35.15) -> (-45.15, 0.15)
  line L23 (-45.15, 0.15) -> (-50.15, 0.15)
  dimension "d137" = 0.15
sketch "Sketch32" plane through (0, 40.5, 0) normal (0, -1, 0) x (1, 0, 0)
  line L0 (-33, 68) -> (-47, 23)
  line L1 (-47, 23) -> (-34.5, 23)
  line L2 (-34.5, 23) -> (-34.5, 35)
  line L3 (-34.5, 35) -> (-31.5, 35)
  line L4 (-31.5, 35) -> (-31.5, 23)
  line L5 (-31.5, 23) -> (-19, 23)
  line L6 (-19, 23) -> (-33, 68) construction
  line L7 (-47.2038, 22.85) -> (-34.35, 22.85)
  line L8 (-34.35, 22.85) -> (-34.35, 34.85)
  line L9 (-34.35, 34.85) -> (-31.65, 34.85)
  line L10 (-31.65, 34.85) -> (-31.65, 22.85)
  line L11 (-31.65, 22.85) -> (-18.7962, 22.85)
  line L12 (-18.7962, 22.85) -> (-33, 68.5049)
  line L13 (-33, 68.5049) -> (-47.2038, 22.85)
  dimension "d138" = 0.15
sketch "Sketch33" plane through (3.5, 0, 0) normal (-1, 0, 0) x (0, -1, 0)
  line L0 (-42.5, 18) -> (-42.5, 23)
  line L1 (-42.5, 23) -> (-44, 23)
  line L2 (-44, 23) -> (-44, 0)
  line L3 (-44, 0) -> (-49, 0)
  line L4 (-49, 0) -> (-49, -5)
  line L5 (-49, -5) -> (-33, -5)
  line L6 (-33, -5) -> (-33, 0)
  line L7 (-33, 0) -> (-38, 0)
  line L8 (-38, 0) -> (-38, 23) construction
  line L9 (-38, 23) -> (-39.5, 23)
  line L10 (-39.5, 23) -> (-39.5, 18)
  line L11 (-39.5, 18) -> (-42.5, 18)
  line L12 (-39.65, 23.15) -> (-39.65, 18.15)
  line L13 (-39.65, 18.15) -> (-42.35, 18.15)
  line L14 (-42.35, 18.15) -> (-42.35, 23.15)
  line L15 (-42.35, 23.15) -> (-44.15, 23.15)
  line L16 (-44.15, 23.15) -> (-44.15, 0.15)
  line L17 (-44.15, 0.15) -> (-49.15, 0.15)
  line L18 (-49.15, 0.15) -> (-49.15, -5.15)
  line L19 (-49.15, -5.15) -> (-32.85, -5.15)
  line L20 (-32.85, -5.15) -> (-32.85, 0.15)
  line L21 (-32.85, 0.15) -> (-37.85, 0.15)
  line L22 (-37.85, 0.15) -> (-37.85, 23.15)
  line L23 (-37.85, 23.15) -> (-39.65, 23.15)
  dimension "d139" = 0.15
sketch "Sketch34" plane through (0, 39.5, 0) normal (0, -1, 0) x (1, 0, 0)
  line L0 (5, 45) -> (-5, 11)
  line L1 (-5, 11) -> (3.5, 11)
  line L2 (3.5, 11) -> (3.5, 23)
  line L3 (3.5, 23) -> (6.5, 23) construction
  line L4 (6.5, 23) -> (6.5, 11)
  line L5 (6.5, 11) -> (15, 11)
  line L6 (15, 11) -> (5, 45)
  line L7 (3.65, 10.85) -> (3.65, 22.85)
  line L8 (3.65, 22.85) -> (6.35, 22.85)
  line L9 (6.35, 22.85) -> (6.35, 10.85)
  line L10 (6.35, 10.85) -> (15.2005, 10.85)
  line L11 (15.2005, 10.85) -> (5, 45.5316)
  line L12 (5, 45.5316) -> (-5.2005, 10.85)
  line L13 (-5.2005, 10.85) -> (3.65, 10.85)
  dimension "d140" = 0.15
extrude "Extrude41" add sketch "Sketch22" along normal blind 1 separate body contours E0 | S0 makes body 18
sketch "Sketch35" plane through (0, 0, 4) normal (0, 0, 1) x (-1, 0, 0)
  line L0 (28.6977, 2.1099) -> (28.6977, -7.5901)
  line L1 (28.6977, -7.5901) -> (25.9977, -7.5901)
  line L2 (25.9977, -7.5901) -> (25.9977, 2.1099)
  line L3 (25.9977, 2.1099) -> (28.6977, 2.1099)
  line L4 (-25.9977, 2.1099) -> (-25.9977, -7.5901)
  line L5 (-25.9977, -7.5901) -> (-28.6977, -7.5901)
  line L6 (-28.6977, -7.5901) -> (-28.6977, 2.1099)
  line L7 (-28.6977, 2.1099) -> (-25.9977, 2.1099)
  line L8 (-3.65, -38.15) -> (-3.65, -43.85)
  line L9 (-3.65, -43.85) -> (-6.35, -43.85)
  line L10 (-6.35, -43.85) -> (-6.35, -38.15)
  line L11 (-6.35, -38.15) -> (-3.65, -38.15)
  line L12 (1.35, -55.15) -> (1.35, -60.85)
  line L13 (1.35, -60.85) -> (-1.35, -60.85)
  line L14 (-1.35, -60.85) -> (-1.35, -55.15)
  line L15 (-1.35, -55.15) -> (1.35, -55.15)
  line L16 (-23.65, -44.15) -> (-23.65, -49.85)
  line L17 (-23.65, -49.85) -> (-26.35, -49.85)
  line L18 (-26.35, -49.85) -> (-26.35, -44.15)
  line L19 (-26.35, -44.15) -> (-23.65, -44.15)
  line L20 (21.35, -47.15) -> (21.35, -52.85)
  line L21 (21.35, -52.85) -> (18.65, -52.85)
  line L22 (18.65, -52.85) -> (18.65, -47.15)
  line L23 (18.65, -47.15) -> (21.35, -47.15)
  line L24 (31.65, -44.85) -> (31.65, -39.15)
  line L25 (31.65, -39.15) -> (34.35, -39.15)
  line L26 (34.35, -39.15) -> (34.35, -44.85)
  line L27 (34.35, -44.85) -> (31.65, -44.85)
  spline S0 degree 3 poles (-50.15, -25) (-50.15, -32.5631) (-47.9958, -40.118) (-43.9509, -46.7448) (-39.8574, -53.4511) (-33.836, -59.192) (-26.6367, -63.255) (-19.363, -67.3601) (-10.9028, -69.7425) (-2.3285, -70.1013) (6.2391, -70.4598) (14.9013, -68.7971) (22.562, -65.3229) (30.4835, -61.7304) (37.313, -56.2069) (42.1269, -49.4968) (46.6731, -43.1599) (49.4152, -35.7814) (50.0195, -28.2553) (50.6245, -20.7198) (49.0848, -13.0525) (45.5885, -6.1855) (42.0575, 0.7493) (36.5382, 6.8528) (29.7144, 11.3714) (22.8186, 15.9376) (14.6055, 18.8748) (6.1105, 19.8136) (-2.4147, 20.7558) (-11.2046, 19.683) (-19.144, 16.731) (-26.9932, 13.8125) (-33.994, 9.0643) (-39.2761, 3.0748) (-44.4865, -2.8334) (-48.014, -9.9366) (-49.4296, -17.3744) (-49.9087, -19.8918) (-50.15, -22.4459) (-50.15, -25) knots -3.141593 -3.141593 -3.141593 -3.141593 -2.639249 -2.639249 -2.639249 -2.130883 -2.130883 -2.130883 -1.617258 -1.617258 -1.617258 -1.10403 -1.10403 -1.10403 -0.573327 -0.573327 -0.573327 -0.072137 -0.072137 -0.072137 0.429687 0.429687 0.429687 0.936474 0.936474 0.936474 1.448612 1.448612 1.448612 1.962576 1.962576 1.962576 2.470707 2.470707 2.470707 2.971946 2.971946 2.971946 3.141593 3.141593 3.141593 3.141593
extrude "Extrude42" add sketch "Sketch23" along normal blind 1 separate body makes body 19
sketch "Sketch36" plane through (-29.8477, 0, 0) normal (-1, 0, 0) x (0, -1, 0)
  line L0 (-5.6188, 25.3335) -> (-7.8901, 23.0621)
  line L1 (-7.8901, 23.0621) -> (-7.8901, 0.1664)
  line L2 (-7.8901, 0.1664) -> (-12.8901, 0.1664)
  line L3 (-12.8901, 0.1664) -> (-12.8901, -5.15)
  line L4 (-12.8901, -5.15) -> (7.4099, -5.15)
  line L5 (7.4099, -5.15) -> (7.4099, 0.1664)
  line L6 (7.4099, 0.1664) -> (2.4099, 0.1664)
  line L7 (2.4099, 0.1664) -> (2.4099, 13.0621)
  line L8 (2.4099, 13.0621) -> (0.3507, 15.1213)
  line L9 (0.3507, 15.1213) -> (2.472, 17.2426)
  line L10 (2.472, 17.2426) -> (-5.6188, 25.3335)
extrude "Extrude43" add sketch "Sketch24" along normal blind 1 separate body makes body 20
sketch "Sketch37" plane through (0, -10.4584, 10.4584) normal (0, -0.707107, 0.707107) x (1, 0, 0)
  line L0 (25.9977, 10.7444) -> (25.9977, 21.5865)
  line L1 (25.9977, 21.5865) -> (28.6977, 21.5865)
  line L2 (28.6977, 21.5865) -> (28.6977, 10.7444)
  line L3 (28.6977, 10.7444) -> (25.9977, 10.7444)
  line L4 (-28.6977, 10.7444) -> (-28.6977, 21.5865)
  line L5 (-28.6977, 21.5865) -> (-25.9977, 21.5865)
  line L6 (-25.9977, 21.5865) -> (-25.9977, 10.7444)
  line L7 (-25.9977, 10.7444) -> (-28.6977, 10.7444)
  arc A0 (-28, 26.1292) -> (-33.15, 20.9792) centre (-28, 20.9792) ccw
  line L8 (-33.15, 20.9792) -> (-33.15, 10.8372)
  arc A1 (-33.15, 10.8372) -> (-28, 5.6872) centre (-28, 10.8372) ccw
  line L9 (-28, 5.6872) -> (28, 5.6872)
  arc A2 (28, 5.6872) -> (33.15, 10.8372) centre (28, 10.8372) ccw
  line L10 (33.15, 10.8372) -> (33.15, 20.9792)
  arc A3 (33.15, 20.9792) -> (28, 26.1292) centre (28, 20.9792) ccw
  line L11 (28, 26.1292) -> (-28, 26.1292)
extrude "Extrude44" add sketch "Sketch25" along normal blind 1 separate body makes body 21
sketch "Sketch38" plane through (-2.5, 0, 0) normal (-1, 0, 0) x (0, -1, 0)
  line L0 (-54.85, 38.15) -> (-56.65, 38.15)
  line L1 (-56.65, 38.15) -> (-56.65, 33.15)
  line L2 (-56.65, 33.15) -> (-59.35, 33.15)
  line L3 (-59.35, 33.15) -> (-59.35, 38.15)
  line L4 (-59.35, 38.15) -> (-61.15, 38.15)
  line L5 (-61.15, 38.15) -> (-61.15, 0.15)
  line L6 (-61.15, 0.15) -> (-66.15, 0.15)
  line L7 (-66.15, 0.15) -> (-66.15, -5.15)
  line L8 (-66.15, -5.15) -> (-49.85, -5.15)
  line L9 (-49.85, -5.15) -> (-49.85, 0.15)
  line L10 (-49.85, 0.15) -> (-54.85, 0.15)
  line L11 (-54.85, 0.15) -> (-54.85, 38.15)
extrude "Extrude45" add sketch "Sketch26" along normal blind 1 separate body makes body 22
sketch "Sketch39" plane through (0, 55.5, 0) normal (0, -1, 0) x (1, 0, 0)
  line L0 (-16.2675, 22.4988) -> (-1.35, 22.4988)
  line L1 (-1.35, 22.4988) -> (-1.35, 37.85)
  line L2 (-1.35, 37.85) -> (1.35, 37.85)
  line L3 (1.35, 37.85) -> (1.35, 22.4988)
  line L4 (1.35, 22.4988) -> (16.2675, 22.4988)
  line L5 (16.2675, 22.4988) -> (0, 70.4671)
  line L6 (0, 70.4671) -> (-16.2675, 22.4988)
extrude "Extrude46" add sketch "Sketch27" along normal blind 1 separate body makes body 23
sketch "Sketch40" plane through (-22.5, 0, 0) normal (-1, 0, 0) x (0, -1, 0)
  line L0 (-53.15, 0.15) -> (-58.15, 0.15)
  line L1 (-58.15, 0.15) -> (-58.15, -5.15)
  line L2 (-58.15, -5.15) -> (-41.85, -5.15)
  line L3 (-41.85, -5.15) -> (-41.85, 0.15)
  line L4 (-41.85, 0.15) -> (-46.85, 0.15)
  line L5 (-46.85, 0.15) -> (-46.85, 28.15)
  line L6 (-46.85, 28.15) -> (-48.65, 28.15)
  line L7 (-48.65, 28.15) -> (-48.65, 23.15)
  line L8 (-48.65, 23.15) -> (-51.35, 23.15)
  line L9 (-51.35, 23.15) -> (-51.35, 28.15)
  line L10 (-51.35, 28.15) -> (-53.15, 28.15)
  line L11 (-53.15, 28.15) -> (-53.15, 0.15)
extrude "Extrude47" add sketch "Sketch28" along normal blind 1 separate body makes body 24
sketch "Sketch41" plane through (0, 47.5, 0) normal (0, -1, 0) x (1, 0, 0)
  line L0 (-34.2132, 15.85) -> (-21.35, 15.85)
  line L1 (-21.35, 15.85) -> (-21.35, 27.85)
  line L2 (-21.35, 27.85) -> (-18.65, 27.85)
  line L3 (-18.65, 27.85) -> (-18.65, 15.85)
  line L4 (-18.65, 15.85) -> (-5.7868, 15.85)
  line L5 (-5.7868, 15.85) -> (-20, 55.444)
  line L6 (-20, 55.444) -> (-34.2132, 15.85)
extrude "Extrude48" add sketch "Sketch29" along normal blind 1 separate body makes body 25
sketch "Sketch42" plane through (22.5, 0, 0) normal (-1, 0, 0) x (0, -1, 0)
  line L0 (-50.15, 0.15) -> (-55.15, 0.15)
  line L1 (-55.15, 0.15) -> (-55.15, -5.15)
  line L2 (-55.15, -5.15) -> (-38.85, -5.15)
  line L3 (-38.85, -5.15) -> (-38.85, 0.15)
  line L4 (-38.85, 0.15) -> (-43.85, 0.15)
  line L5 (-43.85, 0.15) -> (-43.85, 33.15)
  line L6 (-43.85, 33.15) -> (-45.65, 33.15)
  line L7 (-45.65, 33.15) -> (-45.65, 28.15)
  line L8 (-45.65, 28.15) -> (-48.35, 28.15)
  line L9 (-48.35, 28.15) -> (-48.35, 33.15)
  line L10 (-48.35, 33.15) -> (-50.15, 33.15)
  line L11 (-50.15, 33.15) -> (-50.15, 0.15)
extrude "Extrude49" add sketch "Sketch30" along normal blind 1 separate body makes body 26
sketch "Sketch43" plane through (0, 44.5, 0) normal (0, -1, 0) x (1, 0, 0)
  line L0 (9.7919, 19.85) -> (23.65, 19.85)
  line L1 (23.65, 19.85) -> (23.65, 28)
  line L2 (23.65, 28) -> (23.65, 32.85)
  line L3 (23.65, 32.85) -> (26.35, 32.85)
  line L4 (26.35, 32.85) -> (26.35, 28)
  line L5 (26.35, 28) -> (26.35, 19.85)
  line L6 (26.35, 19.85) -> (40.2081, 19.85)
  line L7 (40.2081, 19.85) -> (25, 65.4743)
  line L8 (25, 65.4743) -> (9.7919, 19.85)
extrude "Extrude50" add sketch "Sketch31" along normal blind 1 separate body makes body 27